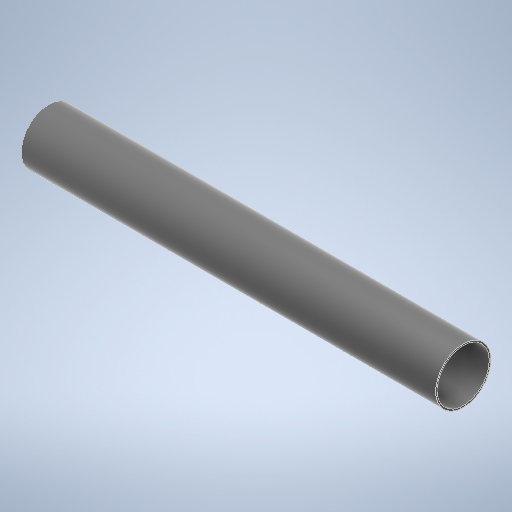
# Autodesk Inventor part: tubo_0002_0001
Saved by Autodesk Inventor 2025.2 (Build 292293000, 293)
## iProperties
Created: 2025-03-25
Part Number: tubo_0002_0001
Material: Thermoplastic Resin
Document SubType Name: Modeling
Designer: kenne
Density: 1.28 g/cm^3
Appearance: Smooth - Black
Author: kenne
Autodesk Inventor part; units mm, degrees
ref_plane "YZ Plane" through (0, 0, 0) normal (1, 0, 0) x (0, 1, 0)
ref_plane "XZ Plane" through (0, 0, 0) normal (0, 1, 0) x (-1, 0, 0)
ref_plane "XY Plane" through (0, 0, 0) normal (0, 0, 1) x (1, 0, 0)
sketch "Sketch1" plane through (0, 0, 0) normal (0, 0, 1) x (1, 0, 0)
  line L0 (-375, 47) -> (375, 47)
  line L1 (375, 47) -> (375, 50)
  line L2 (375, 50) -> (-375, 50)
  line L3 (-375, 50) -> (-375, 47)
  line L4 (-375, 47) -> (375, 50) construction
  line L5 (375, 47) -> (-375, 50) construction
  line L6 (-525, 0) -> (525, 0) projected
  point P0 (0, 0)
  point P1 (0, 48.5)
  point P2 (0, 47)
  dimension "d0" = 750
  dimension "d1" = 3
  dimension "d2" = 50
  constraints: 12 end point, 3 midpoint, 2 parallel, 1 horizontal, 1 perpendicular, 1 vertical alignment
  measures "d0" distance of L2.end L1.end
  measures "d1" distance between parallel lines of L0 L2
  measures "d2" distance from line of point (0, 0) L2
revolve "Revolution1" add sketch "Sketch1" angle 360 about axis through (-10, 0, 0) along (1, 0, 0)
body "Solid1"
